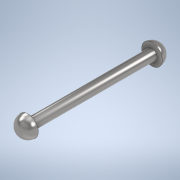
# Autodesk Inventor part: wheelshaft
Saved by Autodesk Inventor 2020.3 (Build 243373000, 373)
## iProperties
Created: 2022-06-23
Part Number: wheelshaft
Material: Stainless Steel, 440C
Document SubType Name: Modeling
Designer: 0x6f736f646f
Density: 7.75 g/cm^3
Appearance: Semi-Polished
Author: 0x6f736f646f
Autodesk Inventor part; units mm, degrees
ref_plane "YZ Plane" through (0, 0, 0) normal (1, 0, 0) x (0, 1, 0)
ref_plane "XZ Plane" through (0, 0, 0) normal (0, 1, 0) x (-1, 0, 0)
ref_plane "XY Plane" through (0, 0, 0) normal (0, 0, 1) x (1, 0, 0)
sketch "Sketch1" plane through (0, 0, 0) normal (1, 0, 0) x (0, 1, 0)
  line L0 (0, 0) -> (2.5, 0)
  line L1 (2.5, 60) -> (0, 60)
  line L2 (0, 60) -> (0, 0)
  arc A0 (2.5, 65) -> (-2.5, 60) centre (2.5, 60) ccw
  arc A1 (-2.5, 0) -> (2.5, -5) centre (2.5, 0) ccw
  line L3 (0, 0) -> (-2.5, 0)
  line L4 (0, 60) -> (-2.5, 60)
  line L5 (2.5, 65) -> (2.5, -5)
  dimension "d1" = 60
  dimension "d2" = 10
  dimension "d3" = 10
  dimension "d5" = 2.5
  dimension "d6" = 70
  constraints: 12 end point, 4 point on circle, 2 centre point, 2 point on line, 1 horizontal, 1 parallel
  measures "d1" distance between parallel lines of L0 L1
  measures "d2" diameter of A0
  measures "d3" diameter of A1
  measures "d5" distance between parallel lines of L2 L5
  measures "d6" distance of L5.start L5.end
revolve "Revolution1" add sketch "Sketch1" angle 360 about axis through (0, 2.5, 65) along (0, 0, -1)
body "Solid1"
